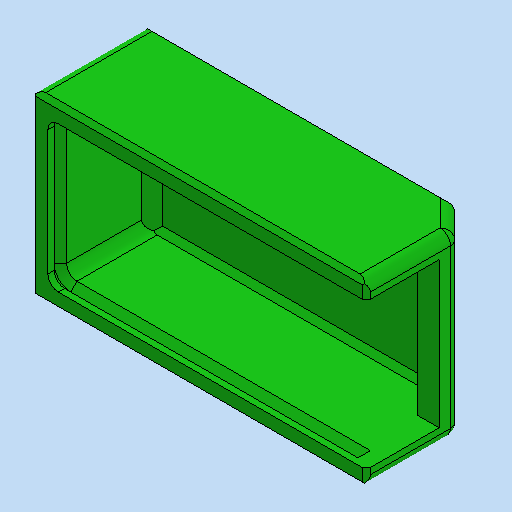
# Autodesk Inventor part: Usbcase-bottom
Saved by Autodesk Inventor 2025 (Build 290162000, 162)
## iProperties
Created: 2025-05-16
Part Number: Usbcase-bottom
Material: ABS Plastic
Document SubType Name: Modeling
Designer: kuzmin
Density: 1.06 g/cm^3
Appearance: Smooth - White
Author: kuzmin
Autodesk Inventor part; units mm, degrees
ref_plane "YZ Plane" through (0, 0, 0) normal (1, 0, 0) x (0, 1, 0)
ref_plane "XZ Plane" through (0, 0, 0) normal (0, 1, 0) x (-1, 0, 0)
ref_plane "XY Plane" through (0, 0, 0) normal (0, 0, 1) x (1, 0, 0)
sketch "Sketch1" plane through (0, 0, 0) normal (0, 0, 1) x (1, 0, 0)
  line L0 (-14.5, 7) -> (14.5, 7)
  line L1 (14.5, 7) -> (14.5, -7)
  line L2 (14.5, -7) -> (-14.5, -7)
  line L3 (-14.5, -7) -> (-14.5, 7)
  line L4 (-16.1, 8.6) -> (16.1, 8.6)
  line L5 (16.1, 8.6) -> (16.1, -8.6)
  line L6 (16.1, -8.6) -> (-16.1, -8.6)
  line L7 (-16.1, -8.6) -> (-16.1, 8.6)
  point P0 (0, 0)
  point P1 (0, 7)
  point P2 (14.5, 0)
  point P3 (0, 8.6)
  point P4 (16.1, 0)
  dimension "d0" = 14
  dimension "d1" = 29
  dimension "d2" = 1.6
  dimension "d3" = 1.6
  constraints: 16 end point, 4 midpoint, 4 parallel, 2 horizontal, 2 horizontal alignment, 2 perpendicular, 2 vertical alignment
  measures "d0" distance of L0.end L1.end
  measures "d1" distance of L0.start L0.end
  measures "d2" distance between parallel lines of L5 L1
  measures "d3" distance between parallel lines of L4 L0
extrude "Extrusion1" add sketch "Sketch1" along normal blind 1 contours L0 L1 L2 L3 | L4 L5 L6 L7
extrude "Extrusion2" add sketch "Sketch1" along normal blind 11
sketch "Sketch2" plane through (0, 0, 11) normal (0, 0, 1) x (1, 0, 0)
  line L0 (16.1, 7) -> (14.5, 7)
  line L1 (14.5, 7) -> (14.5, -7)
  line L2 (14.5, -7) -> (16.1, -7)
  line L3 (16.1, -7) -> (16.1, 7)
  line L4 (14.5, 7) -> (14.5, -7) projected
  line L5 (16.1, -8.6) -> (16.1, 8.6) projected
  point P0 (0, 0)
  point P1 (16.1, 0)
  dimension "d8" = 14
  constraints: 8 end point, 2 parallel, 2 point on line, 1 horizontal, 1 horizontal alignment, 1 midpoint, 1 perpendicular
  measures "d8" distance of L2.end L0.start
extrude "Extrusion3" cut sketch "Sketch2" against normal up to surface (10 mm away)
chamfer "Chamfer1" distance 0.4 angle 45 6 edges at (-16.1, 0, 0) (0, -8.6, 11) (16.1, 7.8, 11) (16.1, -7.8, 11) (-16.1, 0, 11) (0, 8.6, 11)
sketch "Sketch4" plane through (0, 0, 1) normal (0, 0, 1) x (1, 0, 0)
  line L0 (16.1, 7) -> (14, 7)
  line L1 (14, 7) -> (14, -7)
  line L2 (14, -7) -> (16.1, -7)
  line L3 (16.1, -7) -> (16.1, 7)
  line L4 (16.1, 7) -> (16.1, -7) projected
  point P0 (0, 0)
  point P1 (16.1, 0)
  point P2 (16.1, 6.6)
  point P3 (16.1, -6.6)
  dimension "d19" = 2.1
  dimension "d20" = 14
  constraints: 8 end point, 2 midpoint, 2 parallel, 1 horizontal, 1 perpendicular, 1 point on line
  measures "d19" distance between parallel lines of L4 L1
  measures "d20" distance of L2.end L0.start
extrude "Extrusion5" add sketch "Sketch4" along normal blind 3
chamfer "Chamfer10" distance 2.5 angle 45 1 edges at (16.1, 0, 0)
chamfer "Chamfer11" distance 0.4 angle 45 2 edges at (-1.05, -8.6, 0) (-1.05, 8.6, 0)
chamfer "Chamfer16" distance 1 angle 45 1 edges at (-14.5, 0, 1)
chamfer "Chamfer17" distance 0.5 angle 45 2 edges at (0.25, 7, 1) (0.25, -7, 1)
fillet "Fillet14" radius 1 2 edges at (-14.5, -7, 6.5) (-14.5, 7, 6.5)
sketch "Sketch5" plane through (0, 0, 0) normal (1, 0, 0) x (0, 1, 0)
  line L0 (6.7, 10.7) -> (6.7, 8.9)
  line L1 (6.7, 8.9) -> (7.6, 9.8)
  line L2 (7.6, 9.8) -> (6.7, 10.7)
  line L3 (7, 10.6) -> (7, 4) projected
  line L4 (-8.2, 11) -> (8.2, 11) projected
  point P0 (0, 0)
  point P1 (7, 1.4)
  point P2 (-6.5, 11)
  dimension "d24" = 90
  dimension "d30" = 0.9
  dimension "d117" = 0.6
  dimension "d125" = 1.2
  constraints: 6 end point, 1 perpendicular, 1 vertical
  measures "d24" angle of L1 L2
  measures "d30" distance from line of L0 L1.end
  measures "d117" distance from line of L1.end L3
  measures "d125" distance from line of L1.end L4
sketch3d "3D Sketch2"
  line L0 (15.7, 7, 11) -> (-13.5, 7, 11)
  arc A0 (-13.5, 7, 11) -> (-14.5, 6, 11) centre (-13.5, 6, 11) ccw
  line L1 (-14.5, 6, 11) -> (-14.5, -6, 11)
  arc A1 (-14.5, -6, 11) -> (-13.5, -7, 11) centre (-13.5, -6, 11) ccw
  line L2 (-13.5, -7, 11) -> (15.7, -7, 11)
sweep "Sweep2" cut profiles "Sketch5" path "3D Sketch2"
fillet "Fillet4" radius 1 4 edges at (-16.1, -8.6, 5.5) (-16.1, 8.6, 5.5) (16.1, 8.6, 6.55) (16.1, -8.6, 6.55)
sketch "Sketch14" plane through (15.7, 7, 9.2) normal (-1, 0, 0) x (0, 0, 1)
  line L0 (1.2, 0) -> (0, 0) projected
  line L1 (0.6, 0.6) -> (1.2, 0) projected
  line L2 (0, 0) -> (0.6, 0.6) projected
  line L3 (0, -14) -> (1.2, -14) projected
  line L4 (0.6, -14.6) -> (0, -14) projected
  line L5 (1.2, -14) -> (0.6, -14.6) projected
  point P0 (-9.2, -7)
extrude "Extrusion15" add sketch "Sketch14" along normal blind 1
fillet "Fillet15" radius 1 5 edges at (15.8071, -8.3071, 2.2071) (16.1, 0, 2.5) (15.8071, 8.3071, 2.2071) (14.55, 8.6, 0.95) (14.55, -8.6, 0.95)
chamfer "Chamfer18" distance 0.5 angle 45 1 edges at (14, 0, 1)
sketch "Sketch7" plane through (0, 0, 11) normal (0, 0, -1) x (-1, 0, 0)
  line L0 (13.5, -7) -> (-14.7, -7) projected
  line L1 (-16.1, -7) -> (-14, -7) projected
  line L2 (14.5, 6) -> (14.5, -6) projected
  line L3 (-14.7, 7) -> (13.5, 7) projected
  line L4 (-14, 7) -> (-16.1, 7) projected
  line L5 (-16.1, -7) -> (14.5, -7)
  line L6 (14.5, -7) -> (14.5, 7)
  line L7 (14.5, 7) -> (-16.1, 7)
  line L8 (-16.1, 7) -> (-16.1, -7)
  line L9 (14.3, 6.8) -> (14.3, -6.8)
  line L10 (14.3, -6.8) -> (-15.9, -6.8)
  line L11 (-15.9, -6.8) -> (-15.9, 6.8)
  line L12 (-15.9, 6.8) -> (14.3, 6.8)
  line L13 (-15.1, 6) -> (-15.1, -6)
  line L14 (-15.1, -6) -> (13.5, -6)
  line L15 (13.5, -6) -> (13.5, 6)
  line L16 (13.5, 6) -> (-15.1, 6)
  line L17 (13.5, 7) -> (-14.7, 7) projected
  line L18 (14.5, -6) -> (14.5, 6) projected
  line L19 (-14.7, -7) -> (13.5, -7) projected
  line L20 (-14, 7) -> (13.5, 7) projected
  line L21 (-15.7, 7) -> (-16.1, 7) projected
  line L22 (13.5, 7) -> (-15.7, 7) projected
  line L23 (14.5, 6) -> (14.5, -6) projected
  line L24 (14.5, -6) -> (14.5, 6) projected
  line L25 (-15.7, -7) -> (13.5, -7) projected
  line L26 (-16.1, -7) -> (-15.7, -7) projected
  line L27 (13.5, -7) -> (-14, -7) projected
  point P0 (0, 0)
  dimension "d36" = 0.2
  dimension "d37" = 0.8
  constraints: 24 end point, 6 parallel, 3 perpendicular, 2 point on line, 1 horizontal, 6 other
  measures "d36" distance between parallel lines of L8 L11
  measures "d37" distance between parallel lines of L13 L11
sketch "Sketch8" plane through (12, 0, 0) normal (1, 0, 0) x (0, 0, -1)
  line L0 (-9, 6.8) -> (-9.8, 7.6) projected
  line L1 (-9.8, 7.6) -> (-10.6, 6.8) projected
  line L2 (-11, 6.8) -> (-8.8, 6.8) projected
  line L3 (-10.4586, 6.8) -> (-9.8, 7.4586)
  line L4 (-9.8, 7.4586) -> (-9.1414, 6.8)
  line L5 (-8.8, 6.8) -> (-11, 6.8) projected
  line L6 (-9, 6.8) -> (-10.6, 6.8) projected
  point P0 (0, 0)
  point P1 (-10.6, 6.8)
  point P2 (-9, 6.8)
  point P3 (-9, 6.8)
  point P4 (-10.6, 6.8)
  dimension "d49" = 0.1
  constraints: 4 end point, 2 perpendicular, 2 point on line, 1 vertical alignment
  measures "d49" distance between parallel lines of L1 L3
sketch "Sketch9" plane through (0, 0, 12) normal (0, 0, 1) x (1, 0, 0)
  line L0 (-16.1, 14.5689) -> (-6.1, 14.5689)
  line L1 (-6.1, 14.5689) -> (-6.1, -14.5689)
  line L2 (-6.1, -14.5689) -> (-16.1, -14.5689)
  line L3 (-16.1, -14.5689) -> (-16.1, 14.5689)
  line L4 (-16.1, 7.6) -> (-16.1, -7.6) projected
  point P0 (0, 0)
  point P1 (-16.1, 0)
  dimension "d56" = 10
  constraints: 8 end point, 2 midpoint, 2 parallel, 1 horizontal, 1 perpendicular
  measures "d56" distance of L0.start L0.end
sketch "Sketch10" plane through (0, 0, 11) normal (0, 0, -1) x (-1, 0, 0)
  line L0 (-8.1, -6.8) -> (-16.1, -6.8)
  line L1 (-16.1, -6.8) -> (-16.1, 6.8)
  line L2 (-16.1, 6.8) -> (-8.1, 6.8)
  line L3 (-8.1, 6.8) -> (-8.1, -6.8)
  line L4 (-16.1, -7.6) -> (-16.1, 7.6) projected
  line L5 (-13.9, -6.8) -> (6.1, -6.8) projected
  point P0 (0, 0)
  point P1 (-16.1, 0)
  dimension "d63" = 8
  constraints: 8 end point, 2 parallel, 2 point on line, 1 horizontal, 1 horizontal alignment, 1 midpoint, 1 perpendicular
  measures "d63" distance of L0.start L0.end
sketch "Sketch11" plane through (0, 0, 11) normal (0, 0, -1) x (-1, 0, 0)
  line L0 (6.1, -5.5) -> (6.1, 5.5) projected
  line L1 (6.1, -6.8) -> (4.1, -6.8)
  line L2 (4.1, -6.8) -> (4.1, 6.8)
  line L3 (4.1, 6.8) -> (6.1, 6.8)
  line L4 (6.1, 6.8) -> (6.1, -6.8)
  line L5 (6.1, -5.5) -> (-7.1, -5.5) projected
  line L6 (-7.8, -6.8) -> (6.1, -6.8) projected
  point P0 (0, 0)
  point P1 (4.1, 0)
  point P2 (6.1, 5.5)
  dimension "d73" = 2
  constraints: 8 end point, 2 parallel, 2 point on line, 1 horizontal, 1 horizontal alignment, 1 midpoint, 1 perpendicular
  measures "d73" distance of L2.end L3.end
sketch "Sketch12" plane through (0, 0, 8.5) normal (0, 0, -1) x (-1, 0, 0)
  line L0 (-8.1, -6.8) -> (-8.1, -6) projected
  line L1 (-8.1, -6.8) -> (-9.9, -6.8)
  line L2 (-9.9, -6.8) -> (-9.9, 6.8)
  line L3 (-9.9, 6.8) -> (-8.1, 6.8)
  line L4 (-8.1, 6.8) -> (-8.1, -6.8)
  line L5 (-8.1, 6.8) -> (-15.1, 6.8) projected
  point P0 (0, 0)
  dimension "d85" = 1.8
  constraints: 8 end point, 2 parallel, 1 horizontal, 1 perpendicular, 1 point on line
  measures "d85" distance of L0.start L1.end
sketch3d "3D Sketch2"
equation "\"d2\" = wall"
equation "\"d3\" = wall"
equation "\"wall\" = 1.6"
